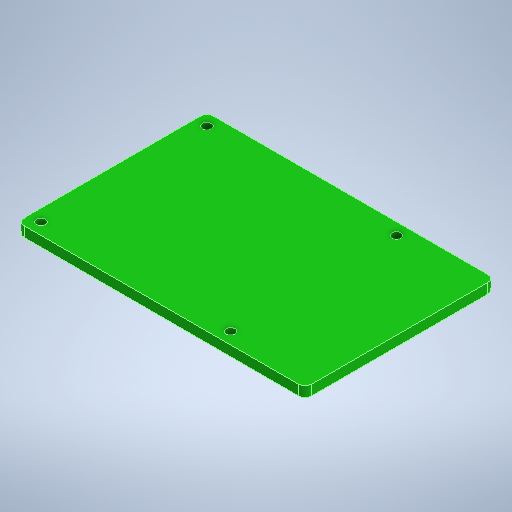
# Autodesk Inventor part: плата двигателей
Saved by Autodesk Inventor 2025 (Build 290162000, 162)
## iProperties
Created: 2025-02-25
Part Number: плата двигателей
Material: Типовые
Document SubType Name: Modeling
Designer: volko
Density: 1 g/cm^3
Appearance: Темно-зеленый
Author: volko
Autodesk Inventor part; units mm, degrees
ref_plane "YZ Plane" through (0, 0, 0) normal (1, 0, 0) x (0, 1, 0)
ref_plane "XZ Plane" through (0, 0, 0) normal (0, 1, 0) x (-1, 0, 0)
ref_plane "XY Plane" through (0, 0, 0) normal (0, 0, 1) x (1, 0, 0)
sketch "Эскиз1" plane through (0, 0, 0) normal (0, 1, 0) x (-1, 0, 0)
  line L0 (40.5, 28) -> (-40.5, 28)
  line L1 (-42.5, 26) -> (-42.5, -26)
  line L2 (-40.5, -28) -> (40.5, -28)
  line L3 (42.5, -26) -> (42.5, 26)
  line L4 (60.0799, 0) -> (-60.0799, 0) projected
  line L5 (0, -39.7799) -> (0, 39.7799) projected
  arc A0 (-40.5, 28) -> (-42.5, 26) centre (-40.5, 26) ccw
  arc A1 (42.5, 26) -> (40.5, 28) centre (40.5, 26) ccw
  arc A2 (40.5, -28) -> (42.5, -26) centre (40.5, -26) ccw
  arc A3 (-42.5, -26) -> (-40.5, -28) centre (-40.5, -26) ccw
  point P0 (0, 0)
  point P1 (42.5, 28)
  point P2 (-42.5, -28)
  point P3 (-42.5, 28)
  point P4 (42.5, -28)
  dimension "d0" = 56
  dimension "d1" = 85
  dimension "d19" = 2
  constraints: 8 end point, 8 point on circle, 8 point on line, 8 tangent, 4 centre point, 3 equal radius, 2 parallel, 1 horizontal, 1 perpendicular, 2 other
  measures "d0" distance between parallel lines of L2 L0
  measures "d1" distance of point (42.5, 28) point (-42.5, 28)
  measures "d19" radius of A0
extrude "Выдавливание1" add sketch "Эскиз1" along normal blind 3
sketch "Эскиз3" plane through (0, 3, 0) normal (0, 1, 0) x (1, 0, 0)
  line L0 (-59.5, 0) -> (59.5, 0) projected
  line L1 (0, 28) -> (0, -28) projected
  line L2 (42.5, -26) -> (42.5, 26) projected
  line L3 (-42.5, 26) -> (-42.5, -26) projected
  point P0 (0, 0)
  point P1 (-39, -24.5)
  point P2 (-39, 24.5)
  point P3 (17, -24.5)
  point P4 (17, 24.5)
  dimension "d13" = 49
  dimension "d16" = 56
  dimension "d21" = 3.5
  constraints: 1 horizontal, 1 symmetric about line, 1 vertical, 3 other
  measures "d13" distance of point (-39, -24.5) point (-39, 24.5)
  measures "d16" distance of point (-39, -24.5) point (17, -24.5)
  measures "d21" distance from line of L3 point (-39, -24.5)
hole "Отверстие1" at (-39, 3, 24.5) at (17, 3, 24.5) at (17, 3, -24.5) at (-39, 3, -24.5) direction (0, -1, 0) diameter 2.7 end through all
